Autodesk Fusion 360 part; units mm, degrees
note: some values were not read from the file. Chosen so that the rebuilt part matches the saved one: a direction. Set by a fixed rule: which sketch regions a step uses.
(part 3 of 8)
  spline S31 degree 5 poles (2.8779, -27.5468) (2.8797, -27.5528) (2.8833, -27.5648) (2.8888, -27.5828) (2.8962, -27.6068) (2.9055, -27.6366) (2.915, -27.6664) (2.9246, -27.6961) (2.9342, -27.7257) (2.944, -27.7552) (2.954, -27.7847) (2.964, -27.814) (2.9742, -27.8433) (2.9845, -27.8725) (2.9949, -27.9015) (3.0054, -27.9305) (3.0161, -27.9594) (3.0268, -27.9882) (3.0377, -28.017) (3.0487, -28.0456) (3.0599, -28.0741) (3.0711, -28.1025) (3.0825, -28.1309) (3.094, -28.1591) (3.1057, -28.1872) (3.1174, -28.2153) (3.1293, -28.2432) (3.1413, -28.271) (3.1535, -28.2987) (3.1657, -28.3264) (3.1781, -28.3539) (3.1907, -28.3813) (3.2033, -28.4086) (3.2161, -28.4357) (3.229, -28.4628) (3.2421, -28.4897) (3.2553, -28.5166) (3.2686, -28.5433) (3.2821, -28.5699) (3.2957, -28.5964) (3.3094, -28.6227) (3.3233, -28.6489) (3.3373, -28.675) (3.3515, -28.701) (3.3658, -28.7268) (3.3802, -28.7525) (3.3948, -28.7781) (3.4096, -28.8035) (3.4244, -28.8288) (3.4395, -28.854) (3.4547, -28.879) (3.47, -28.9038) (3.4856, -28.9285) (3.5013, -28.953) (3.5172, -28.9774) (3.5332, -29.0015) (3.5494, -29.0256) (3.5657, -29.0495) (3.5822, -29.0732) (3.5989, -29.0967) (3.6158, -29.12) (3.6329, -29.1431) (3.6504, -29.1659) (3.668, -29.1884) (3.686, -29.2107) (3.704, -29.2327) (3.7222, -29.2547) (3.7405, -29.2765) (3.759, -29.2981) (3.7779, -29.3193) (3.7972, -29.34) (3.8133, -29.3559) (3.8258, -29.3673) (3.8344, -29.3748) (3.8387, -29.3784) knots -1 -1 -1 -1 -1 -1 -0.98571429 -0.97142857 -0.95714286 -0.94285714 -0.92857143 -0.91428571 -0.9 -0.88571429 -0.87142857 -0.85714286 -0.84285714 -0.82857143 -0.81428571 -0.8 -0.78571429 -0.77142857 -0.75714286 -0.74285714 -0.72857143 -0.71428571 -0.7 -0.68571429 -0.67142857 -0.65714286 -0.64285714 -0.62857143 -0.61428571 -0.6 -0.58571429 -0.57142857 -0.55714286 -0.54285714 -0.52857143 -0.51428571 -0.5 -0.48571429 -0.47142857 -0.45714286 -0.44285714 -0.42857143 -0.41428571 -0.4 -0.38571429 -0.37142857 -0.35714286 -0.34285714 -0.32857143 -0.31428571 -0.3 -0.28571429 -0.27142857 -0.25714286 -0.24285714 -0.22857143 -0.21428571 -0.2 -0.18571429 -0.17142857 -0.15714286 -0.14285714 -0.12857143 -0.11428571 -0.1 -0.08571429 -0.07142857 -0.05714286 -0.04285714 -0.02857143 -0.01428571 0 0 0 0 0 0
  line L31 (3.8387, -29.3784) -> (4.1341, -29.6298)
  arc A63 (4.146, -29.7701) -> (4.1341, -29.6298) centre (4.0693, -29.706) ccw
  arc A64 (4.146, -29.7701) -> (3.5162, -30.5908) centre (13.5, -37.5997) ccw
  arc A65 (3.3776, -30.6157) -> (3.5162, -30.5908) centre (3.4344, -30.5334) ccw
  line L32 (3.3776, -30.6157) -> (3.0583, -30.3954)
  spline S32 degree 5 poles (3.0583, -30.3954) (3.0537, -30.3922) (3.0443, -30.3859) (3.03, -30.3768) (3.0105, -30.3653) (2.9855, -30.352) (2.9601, -30.3393) (2.9345, -30.327) (2.9087, -30.315) (2.8827, -30.3031) (2.8567, -30.2913) (2.8306, -30.2798) (2.8043, -30.2685) (2.7778, -30.2576) (2.751, -30.247) (2.7242, -30.2367) (2.6971, -30.2267) (2.6699, -30.2169) (2.6426, -30.2073) (2.6152, -30.1979) (2.5877, -30.1887) (2.5601, -30.1796) (2.5323, -30.1708) (2.5045, -30.1622) (2.4765, -30.1538) (2.4484, -30.1456) (2.4202, -30.1375) (2.392, -30.1297) (2.3636, -30.1221) (2.3351, -30.1146) (2.3065, -30.1073) (2.2779, -30.1001) (2.2491, -30.0932) (2.2203, -30.0864) (2.1914, -30.0798) (2.1624, -30.0733) (2.1333, -30.067) (2.1041, -30.0609) (2.0748, -30.055) (2.0455, -30.0492) (2.0161, -30.0435) (1.9866, -30.0381) (1.957, -30.0327) (1.9274, -30.0276) (1.8977, -30.0226) (1.8679, -30.0177) (1.8381, -30.013) (1.8082, -30.0085) (1.7782, -30.0041) (1.7481, -29.9998) (1.718, -29.9957) (1.6878, -29.9917) (1.6576, -29.9879) (1.6272, -29.9843) (1.5969, -29.9807) (1.5664, -29.9774) (1.5359, -29.9741) (1.5054, -29.971) (1.4748, -29.9681) (1.4441, -29.9653) (1.4134, -29.9626) (1.3826, -29.9601) (1.3517, -29.9577) (1.3208, -29.9555) (1.2899, -29.9534) (1.2589, -29.9514) (1.2278, -29.9496) (1.1967, -29.9479) (1.1656, -29.9463) (1.1343, -29.9449) (1.1031, -29.9436) (1.078, -29.9427) (1.0592, -29.942) (1.0467, -29.9416) (1.0404, -29.9415) knots 0 0 0 0 0 0 0.01428571 0.02857143 0.04285714 0.05714286 0.07142857 0.08571429 0.1 0.11428571 0.12857143 0.14285714 0.15714286 0.17142857 0.18571429 0.2 0.21428571 0.22857143 0.24285714 0.25714286 0.27142857 0.28571429 0.3 0.31428571 0.32857143 0.34285714 0.35714286 0.37142857 0.38571429 0.4 0.41428571 0.42857143 0.44285714 0.45714286 0.47142857 0.48571429 0.5 0.51428571 0.52857143 0.54285714 0.55714286 0.57142857 0.58571429 0.6 0.61428571 0.62857143 0.64285714 0.65714286 0.67142857 0.68571429 0.7 0.71428571 0.72857143 0.74285714 0.75714286 0.77142857 0.78571429 0.8 0.81428571 0.82857143 0.84285714 0.85714286 0.87142857 0.88571429 0.9 0.91428571 0.92857143 0.94285714 0.95714286 0.97142857 0.98571429 1 1 1 1 1 1
  arc A66 (1.0404, -29.9415) -> (0.638, -30.6385) centre (13.5, -37.5997) ccw
  spline S33 degree 5 poles (0.638, -30.6385) (0.6413, -30.6439) (0.6479, -30.6545) (0.6578, -30.6705) (0.6711, -30.6917) (0.6879, -30.7182) (0.7047, -30.7445) (0.7217, -30.7707) (0.7387, -30.7968) (0.7558, -30.8228) (0.773, -30.8486) (0.7903, -30.8744) (0.8077, -30.9) (0.8252, -30.9255) (0.8428, -30.9509) (0.8604, -30.9762) (0.8782, -31.0014) (0.8961, -31.0264) (0.914, -31.0513) (0.9321, -31.0761) (0.9502, -31.1008) (0.9684, -31.1253) (0.9868, -31.1498) (1.0052, -31.174) (1.0237, -31.1982) (1.0423, -31.2222) (1.061, -31.2461) (1.0798, -31.2699) (1.0988, -31.2935) (1.1178, -31.317) (1.1368, -31.3404) (1.156, -31.3636) (1.1753, -31.3867) (1.1947, -31.4096) (1.2142, -31.4324) (1.2338, -31.4551) (1.2535, -31.4776) (1.2733, -31.5) (1.2931, -31.5222) (1.3131, -31.5442) (1.3332, -31.5661) (1.3534, -31.5879) (1.3737, -31.6094) (1.3941, -31.6309) (1.4146, -31.6521) (1.4352, -31.6732) (1.4559, -31.6941) (1.4768, -31.7149) (1.4977, -31.7355) (1.5187, -31.7559) (1.5399, -31.7761) (1.5611, -31.7961) (1.5825, -31.8159) (1.6041, -31.8355) (1.6257, -31.8549) (1.6474, -31.8741) (1.6693, -31.8931) (1.6913, -31.912) (1.7133, -31.9306) (1.7355, -31.9491) (1.7579, -31.9672) (1.7804, -31.985) (1.8031, -32.0025) (1.826, -32.0197) (1.8491, -32.0366) (1.8723, -32.0532) (1.8955, -32.0697) (1.9189, -32.086) (1.9423, -32.1021) (1.966, -32.1178) (1.9901, -32.1327) (2.0097, -32.1439) (2.0248, -32.1517) (2.0349, -32.1567) (2.04, -32.1591) knots -1 -1 -1 -1 -1 -1 -0.98571429 -0.97142857 -0.95714286 -0.94285714 -0.92857143 -0.91428571 -0.9 -0.88571429 -0.87142857 -0.85714286 -0.84285714 -0.82857143 -0.81428571 -0.8 -0.78571429 -0.77142857 -0.75714286 -0.74285714 -0.72857143 -0.71428571 -0.7 -0.68571429 -0.67142857 -0.65714286 -0.64285714 -0.62857143 -0.61428571 -0.6 -0.58571429 -0.57142857 -0.55714286 -0.54285714 -0.52857143 -0.51428571 -0.5 -0.48571429 -0.47142857 -0.45714286 -0.44285714 -0.42857143 -0.41428571 -0.4 -0.38571429 -0.37142857 -0.35714286 -0.34285714 -0.32857143 -0.31428571 -0.3 -0.28571429 -0.27142857 -0.25714286 -0.24285714 -0.22857143 -0.21428571 -0.2 -0.18571429 -0.17142857 -0.15714286 -0.14285714 -0.12857143 -0.11428571 -0.1 -0.08571429 -0.07142857 -0.05714286 -0.04285714 -0.02857143 -0.01428571 0 0 0 0 0 0
  line L33 (2.04, -32.1591) -> (2.3904, -32.3255)
  arc A67 (2.4382, -32.4579) -> (2.3904, -32.3255) centre (2.3476, -32.4158) ccw
  arc A68 (2.4382, -32.4579) -> (2.0424, -33.4137) centre (13.5, -37.5997) ccw
  arc A69 (1.9149, -33.4735) -> (2.0424, -33.4137) centre (1.9484, -33.3793) ccw
  line L34 (1.9149, -33.4735) -> (1.5495, -33.3434)
  spline S34 degree 5 poles (1.5495, -33.3434) (1.5442, -33.3415) (1.5335, -33.3378) (1.5173, -33.3328) (1.4955, -33.3267) (1.4679, -33.3203) (1.4401, -33.3146) (1.4122, -33.3094) (1.3841, -33.3044) (1.356, -33.2996) (1.3278, -33.295) (1.2996, -33.2907) (1.2713, -33.2866) (1.2428, -33.2829) (1.2143, -33.2796) (1.1856, -33.2766) (1.1569, -33.2739) (1.1281, -33.2715) (1.0993, -33.2693) (1.0704, -33.2673) (1.0414, -33.2655) (1.0124, -33.2639) (0.9833, -33.2626) (0.9542, -33.2615) (0.925, -33.2606) (0.8957, -33.2599) (0.8664, -33.2595) (0.8371, -33.2592) (0.8077, -33.2592) (0.7782, -33.2593) (0.7488, -33.2597) (0.7192, -33.2602) (0.6897, -33.2609) (0.66, -33.2618) (0.6304, -33.2629) (0.6007, -33.2642) (0.571, -33.2656) (0.5412, -33.2673) (0.5114, -33.2691) (0.4816, -33.2711) (0.4517, -33.2733) (0.4218, -33.2756) (0.3919, -33.2781) (0.3619, -33.2808) (0.3319, -33.2836) (0.3019, -33.2867) (0.2719, -33.2898) (0.2418, -33.2932) (0.2117, -33.2967) (0.1815, -33.3004) (0.1514, -33.3042) (0.1212, -33.3082) (0.091, -33.3123) (0.0608, -33.3166) (0.0305, -33.3211) (0.0002, -33.3257) (-0.03, -33.3305) (-0.0604, -33.3354) (-0.0907, -33.3405) (-0.1211, -33.3457) (-0.1514, -33.3511) (-0.1818, -33.3566) (-0.2122, -33.3623) (-0.2427, -33.3681) (-0.2731, -33.3741) (-0.3036, -33.3802) (-0.334, -33.3865) (-0.3645, -33.3929) (-0.395, -33.3995) (-0.4255, -33.4062) (-0.4561, -33.413) (-0.4805, -33.4186) (-0.4988, -33.4229) (-0.511, -33.4257) (-0.5172, -33.4272) knots 0 0 0 0 0 0 0.01428571 0.02857143 0.04285714 0.05714286 0.07142857 0.08571429 0.1 0.11428571 0.12857143 0.14285714 0.15714286 0.17142857 0.18571429 0.2 0.21428571 0.22857143 0.24285714 0.25714286 0.27142857 0.28571429 0.3 0.31428571 0.32857143 0.34285714 0.35714286 0.37142857 0.38571429 0.4 0.41428571 0.42857143 0.44285714 0.45714286 0.47142857 0.48571429 0.5 0.51428571 0.52857143 0.54285714 0.55714286 0.57142857 0.58571429 0.6 0.61428571 0.62857143 0.64285714 0.65714286 0.67142857 0.68571429 0.7 0.71428571 0.72857143 0.74285714 0.75714286 0.77142857 0.78571429 0.8 0.81428571 0.82857143 0.84285714 0.85714286 0.87142857 0.88571429 0.9 0.91428571 0.92857143 0.94285714 0.95714286 0.97142857 0.98571429 1 1 1 1 1 1
  arc A70 (-0.5172, -33.4272) -> (-0.7255, -34.2047) centre (13.5, -37.5997) ccw
  spline S35 degree 5 poles (-0.7255, -34.2047) (-0.7209, -34.209) (-0.7118, -34.2176) (-0.698, -34.2304) (-0.6796, -34.2475) (-0.6566, -34.2687) (-0.6336, -34.2897) (-0.6104, -34.3107) (-0.5872, -34.3315) (-0.564, -34.3521) (-0.5406, -34.3726) (-0.5173, -34.393) (-0.4938, -34.4133) (-0.4703, -34.4334) (-0.4468, -34.4534) (-0.4232, -34.4733) (-0.3995, -34.493) (-0.3758, -34.5125) (-0.352, -34.5319) (-0.3281, -34.5512) (-0.3042, -34.5704) (-0.2803, -34.5894) (-0.2562, -34.6082) (-0.2321, -34.6269) (-0.208, -34.6454) (-0.1838, -34.6638) (-0.1595, -34.6821) (-0.1352, -34.7002) (-0.1108, -34.7181) (-0.0864, -34.7359) (-0.0619, -34.7535) (-0.0374, -34.771) (-0.0128, -34.7883) (0.0119, -34.8054) (0.0366, -34.8224) (0.0614, -34.8392) (0.0862, -34.8558) (0.1111, -34.8723) (0.1361, -34.8886) (0.1611, -34.9048) (0.1862, -34.9207) (0.2113, -34.9365) (0.2365, -34.9521) (0.2618, -34.9675) (0.2871, -34.9827) (0.3124, -34.9977) (0.3379, -35.0126) (0.3633, -35.0272) (0.3889, -35.0417) (0.4145, -35.056) (0.4401, -35.07) (0.4659, -35.0838) (0.4917, -35.0974) (0.5175, -35.1108) (0.5434, -35.124) (0.5694, -35.1369) (0.5954, -35.1496) (0.6215, -35.1621) (0.6477, -35.1744) (0.6739, -35.1865) (0.7002, -35.1982) (0.7266, -35.2096) (0.753, -35.2206) (0.7796, -35.2313) (0.8063, -35.2416) (0.833, -35.2517) (0.8597, -35.2616) (0.8865, -35.2713) (0.9133, -35.2808) (0.9402, -35.2898) (0.9673, -35.298) (0.9892, -35.3037) (1.0057, -35.3073) (1.0168, -35.3095) (1.0224, -35.3105) knots -1 -1 -1 -1 -1 -1 -0.98571429 -0.97142857 -0.95714286 -0.94285714 -0.92857143 -0.91428571 -0.9 -0.88571429 -0.87142857 -0.85714286 -0.84285714 -0.82857143 -0.81428571 -0.8 -0.78571429 -0.77142857 -0.75714286 -0.74285714 -0.72857143 -0.71428571 -0.7 -0.68571429 -0.67142857 -0.65714286 -0.64285714 -0.62857143 -0.61428571 -0.6 -0.58571429 -0.57142857 -0.55714286 -0.54285714 -0.52857143 -0.51428571 -0.5 -0.48571429 -0.47142857 -0.45714286 -0.44285714 -0.42857143 -0.41428571 -0.4 -0.38571429 -0.37142857 -0.35714286 -0.34285714 -0.32857143 -0.31428571 -0.3 -0.28571429 -0.27142857 -0.25714286 -0.24285714 -0.22857143 -0.21428571 -0.2 -0.18571429 -0.17142857 -0.15714286 -0.14285714 -0.12857143 -0.11428571 -0.1 -0.08571429 -0.07142857 -0.05714286 -0.04285714 -0.02857143 -0.01428571 0 0 0 0 0 0
  line L35 (1.0224, -35.3105) -> (1.4039, -35.3805)
  arc A71 (1.4844, -35.4961) -> (1.4039, -35.3805) centre (1.3859, -35.4789) ccw
  arc A72 (1.4844, -35.4961) -> (1.3493, -36.5217) centre (13.5, -37.5997) ccw
  arc A73 (1.2417, -36.6126) -> (1.3493, -36.5217) centre (1.2497, -36.5129) ccw
  line L36 (1.2417, -36.6126) -> (0.8551, -36.5815)
  spline S36 degree 5 poles (0.8551, -36.5815) (0.8494, -36.581) (0.8382, -36.5802) (0.8212, -36.5795) (0.7986, -36.5793) (0.7703, -36.5802) (0.742, -36.5819) (0.7136, -36.5841) (0.6853, -36.5866) (0.6569, -36.5893) (0.6285, -36.5921) (0.6001, -36.5952) (0.5716, -36.5986) (0.5432, -36.6024) (0.5148, -36.6066) (0.4863, -36.6111) (0.4579, -36.6159) (0.4295, -36.6211) (0.401, -36.6264) (0.3726, -36.632) (0.3441, -36.6377) (0.3157, -36.6437) (0.2873, -36.6499) (0.2588, -36.6564) (0.2304, -36.6631) (0.202, -36.67) (0.1736, -36.6772) (0.1451, -36.6845) (0.1167, -36.6921) (0.0883, -36.6999) (0.0599, -36.7078) (0.0316, -36.716) (0.0032, -36.7243) (-0.0252, -36.7328) (-0.0535, -36.7416) (-0.0819, -36.7505) (-0.1102, -36.7596) (-0.1385, -36.7689) (-0.1669, -36.7784) (-0.1952, -36.788) (-0.2234, -36.7978) (-0.2517, -36.8078) (-0.28, -36.818) (-0.3082, -36.8283) (-0.3365, -36.8389) (-0.3647, -36.8495) (-0.3929, -36.8604) (-0.4211, -36.8714) (-0.4492, -36.8826) (-0.4774, -36.8939) (-0.5055, -36.9054) (-0.5337, -36.9171) (-0.5618, -36.9289) (-0.5898, -36.9409) (-0.6179, -36.9531) (-0.646, -36.9653) (-0.674, -36.9778) (-0.702, -36.9904) (-0.73, -37.0032) (-0.7579, -37.0161) (-0.7859, -37.0291) (-0.8138, -37.0423) (-0.8417, -37.0557) (-0.8696, -37.0692) (-0.8975, -37.0828) (-0.9253, -37.0966) (-0.9531, -37.1106) (-0.9809, -37.1247) (-1.0087, -37.1389) (-1.0364, -37.1533) (-1.0641, -37.1678) (-1.0863, -37.1795) (-1.1029, -37.1884) (-1.1139, -37.1943) (-1.1195, -37.1973) knots 0 0 0 0 0 0 0.01428571 0.02857143 0.04285714 0.05714286 0.07142857 0.08571429 0.1 0.11428571 0.12857143 0.14285714 0.15714286 0.17142857 0.18571429 0.2 0.21428571 0.22857143 0.24285714 0.25714286 0.27142857 0.28571429 0.3 0.31428571 0.32857143 0.34285714 0.35714286 0.37142857 0.38571429 0.4 0.41428571 0.42857143 0.44285714 0.45714286 0.47142857 0.48571429 0.5 0.51428571 0.52857143 0.54285714 0.55714286 0.57142857 0.58571429 0.6 0.61428571 0.62857143 0.64285714 0.65714286 0.67142857 0.68571429 0.7 0.71428571 0.72857143 0.74285714 0.75714286 0.77142857 0.78571429 0.8 0.81428571 0.82857143 0.84285714 0.85714286 0.87142857 0.88571429 0.9 0.91428571 0.92857143 0.94285714 0.95714286 0.97142857 0.98571429 1 1 1 1 1 1
  arc A74 (-1.1195, -37.1973) -> (-1.1195, -38.0022) centre (13.5, -37.5997) ccw
  spline S37 degree 5 poles (-1.1195, -38.0022) (-1.1139, -38.0051) (-1.1029, -38.0111) (-1.0863, -38.0199) (-1.0641, -38.0317) (-1.0364, -38.0462) (-1.0087, -38.0605) (-0.9809, -38.0748) (-0.9531, -38.0889) (-0.9253, -38.1028) (-0.8975, -38.1166) (-0.8696, -38.1302) (-0.8417, -38.1437) (-0.8138, -38.1571) (-0.7859, -38.1703) (-0.7579, -38.1834) (-0.73, -38.1963) (-0.702, -38.209) (-0.674, -38.2216) (-0.646, -38.2341) (-0.6179, -38.2464) (-0.5898, -38.2585) (-0.5618, -38.2705) (-0.5337, -38.2823) (-0.5055, -38.294) (-0.4774, -38.3055) (-0.4492, -38.3168) (-0.4211, -38.328) (-0.3929, -38.339) (-0.3647, -38.3499) (-0.3365, -38.3606) (-0.3082, -38.3711) (-0.28, -38.3814) (-0.2517, -38.3916) (-0.2234, -38.4016) (-0.1952, -38.4114) (-0.1669, -38.4211) (-0.1385, -38.4305) (-0.1102, -38.4398) (-0.0819, -38.4489) (-0.0535, -38.4579) (-0.0252, -38.4666) (0.0032, -38.4751) (0.0316, -38.4835) (0.0599, -38.4916) (0.0883, -38.4996) (0.1167, -38.5073) (0.1451, -38.5149) (0.1736, -38.5223) (0.202, -38.5294) (0.2304, -38.5364) (0.2588, -38.5431) (0.2873, -38.5495) (0.3157, -38.5557) (0.3441, -38.5617) (0.3726, -38.5675) (0.401, -38.573) (0.4295, -38.5784) (0.4579, -38.5835) (0.4863, -38.5883) (0.5148, -38.5929) (0.5432, -38.5971) (0.5716, -38.6008) (0.6001, -38.6043) (0.6285, -38.6073) (0.6569, -38.6102) (0.6853, -38.6128) (0.7136, -38.6153) (0.742, -38.6175) (0.7703, -38.6192) (0.7986, -38.6201) (0.8212, -38.6199) (0.8382, -38.6192) (0.8494, -38.6184) (0.8551, -38.618) knots -1 -1 -1 -1 -1 -1 -0.98571429 -0.97142857 -0.95714286 -0.94285714 -0.92857143 -0.91428571 -0.9 -0.88571429 -0.87142857 -0.85714286 -0.84285714 -0.82857143 -0.81428571 -0.8 -0.78571429 -0.77142857 -0.75714286 -0.74285714 -0.72857143 -0.71428571 -0.7 -0.68571429 -0.67142857 -0.65714286 -0.64285714 -0.62857143 -0.61428571 -0.6 -0.58571429 -0.57142857 -0.55714286 -0.54285714 -0.52857143 -0.51428571 -0.5 -0.48571429 -0.47142857 -0.45714286 -0.44285714 -0.42857143 -0.41428571 -0.4 -0.38571429 -0.37142857 -0.35714286 -0.34285714 -0.32857143 -0.31428571 -0.3 -0.28571429 -0.27142857 -0.25714286 -0.24285714 -0.22857143 -0.21428571 -0.2 -0.18571429 -0.17142857 -0.15714286 -0.14285714 -0.12857143 -0.11428571 -0.1 -0.08571429 -0.07142857 -0.05714286 -0.04285714 -0.02857143 -0.01428571 0 0 0 0 0 0
  line L37 (0.8551, -38.618) -> (1.2417, -38.5868)
  arc A75 (1.3493, -38.6777) -> (1.2417, -38.5868) centre (1.2497, -38.6865) ccw
  arc A76 (1.3493, -38.6777) -> (1.4844, -39.7033) centre (13.5, -37.5997) ccw
  arc A77 (1.4039, -39.8189) -> (1.4844, -39.7033) centre (1.3859, -39.7205) ccw
  line L38 (1.4039, -39.8189) -> (1.0224, -39.8889)
  spline S38 degree 5 poles (1.0224, -39.8889) (1.0168, -39.8899) (1.0057, -39.8921) (0.9892, -39.8958) (0.9673, -39.9015) (0.9402, -39.9097) (0.9133, -39.9186) (0.8865, -39.9281) (0.8597, -39.9378) (0.833, -39.9477) (0.8063, -39.9578) (0.7796, -39.9682) (0.753, -39.9788) (0.7266, -39.9898) (0.7002, -40.0012) (0.6739, -40.013) (0.6477, -40.025) (0.6215, -40.0373) (0.5954, -40.0498) (0.5694, -40.0626) (0.5434, -40.0755) (0.5175, -40.0886) (0.4917, -40.102) (0.4659, -40.1156) (0.4401, -40.1294) (0.4145, -40.1435) (0.3889, -40.1577) (0.3633, -40.1722) (0.3379, -40.1869) (0.3124, -40.2017) (0.2871, -40.2167) (0.2618, -40.232) (0.2365, -40.2474) (0.2113, -40.2629) (0.1862, -40.2787) (0.1611, -40.2947) (0.1361, -40.3108) (0.1111, -40.3271) (0.0862, -40.3436) (0.0614, -40.3602) (0.0366, -40.377) (0.0119, -40.394) (-0.0128, -40.4112) (-0.0374, -40.4285) (-0.0619, -40.4459) (-0.0864, -40.4636) (-0.1108, -40.4813) (-0.1352, -40.4993) (-0.1595, -40.5174) (-0.1838, -40.5356) (-0.208, -40.554) (-0.2321, -40.5725) (-0.2562, -40.5912) (-0.2803, -40.6101) (-0.3042, -40.6291) (-0.3281, -40.6482) (-0.352, -40.6675) (-0.3758, -40.6869) (-0.3995, -40.7065) (-0.4232, -40.7262) (-0.4468, -40.746) (-0.4703, -40.766) (-0.4938, -40.7861) (-0.5173, -40.8064) (-0.5406, -40.8268) (-0.564, -40.8473) (-0.5872, -40.868) (-0.6104, -40.8888) (-0.6336, -40.9097) (-0.6566, -40.9308) (-0.6796, -40.952) (-0.698, -40.969) (-0.7118, -40.9819) (-0.7209, -40.9905) (-0.7255, -40.9948) knots 0 0 0 0 0 0 0.01428571 0.02857143 0.04285714 0.05714286 0.07142857 0.08571429 0.1 0.11428571 0.12857143 0.14285714 0.15714286 0.17142857 0.18571429 0.2 0.21428571 0.22857143 0.24285714 0.25714286 0.27142857 0.28571429 0.3 0.31428571 0.32857143 0.34285714 0.35714286 0.37142857 0.38571429 0.4 0.41428571 0.42857143 0.44285714 0.45714286 0.47142857 0.48571429 0.5 0.51428571 0.52857143 0.54285714 0.55714286 0.57142857 0.58571429 0.6 0.61428571 0.62857143 0.64285714 0.65714286 0.67142857 0.68571429 0.7 0.71428571 0.72857143 0.74285714 0.75714286 0.77142857 0.78571429 0.8 0.81428571 0.82857143 0.84285714 0.85714286 0.87142857 0.88571429 0.9 0.91428571 0.92857143 0.94285714 0.95714286 0.97142857 0.98571429 1 1 1 1 1 1
  arc A78 (-0.7255, -40.9948) -> (-0.5172, -41.7722) centre (13.5, -37.5997) ccw
  spline S39 degree 5 poles (-0.5172, -41.7722) (-0.511, -41.7737) (-0.4988, -41.7766) (-0.4805, -41.7808) (-0.4561, -41.7864) (-0.4255, -41.7933) (-0.395, -41.8) (-0.3645, -41.8065) (-0.334, -41.8129) (-0.3036, -41.8192) (-0.2731, -41.8253) (-0.2427, -41.8313) (-0.2122, -41.8371) (-0.1818, -41.8428) (-0.1514, -41.8483) (-0.1211, -41.8537) (-0.0907, -41.8589) (-0.0604, -41.864) (-0.03, -41.8689) (0.0002, -41.8737) (0.0305, -41.8783) (0.0608, -41.8828) (0.091, -41.8871) (0.1212, -41.8912) (0.1514, -41.8952) (0.1815, -41.8991) (0.2117, -41.9027) (0.2418, -41.9062) (0.2719, -41.9096) (0.3019, -41.9128) (0.3319, -41.9158) (0.3619, -41.9186) (0.3919, -41.9213) (0.4218, -41.9238) (0.4517, -41.9262) (0.4816, -41.9283) (0.5114, -41.9303) (0.5412, -41.9321) (0.571, -41.9338) (0.6007, -41.9353) (0.6304, -41.9365) (0.66, -41.9376) (0.6897, -41.9385) (0.7192, -41.9393) (0.7488, -41.9398) (0.7782, -41.9401) (0.8077, -41.9403) (0.8371, -41.9402) (0.8664, -41.94) (0.8957, -41.9395) (0.925, -41.9389) (0.9542, -41.938) (0.9833, -41.9369) (1.0124, -41.9355) (1.0414, -41.9339) (1.0704, -41.9321) (1.0993, -41.9301) (1.1281, -41.9279) (1.1569, -41.9255) (1.1856, -41.9228) (1.2143, -41.9199) (1.2428, -41.9165) (1.2713, -41.9128) (1.2996, -41.9088) (1.3278, -41.9044) (1.356, -41.8998) (1.3841, -41.895) (1.4122, -41.89) (1.4401, -41.8848) (1.4679, -41.8791) (1.4955, -41.8727) (1.5173, -41.8667) (1.5335, -41.8616) (1.5442, -41.8579) (1.5495, -41.856) knots -1 -1 -1 -1 -1 -1 -0.98571429 -0.97142857 -0.95714286 -0.94285714 -0.92857143 -0.91428571 -0.9 -0.88571429 -0.87142857 -0.85714286 -0.84285714 -0.82857143 -0.81428571 -0.8 -0.78571429 -0.77142857 -0.75714286 -0.74285714 -0.72857143 -0.71428571 -0.7 -0.68571429 -0.67142857 -0.65714286 -0.64285714 -0.62857143 -0.61428571 -0.6 -0.58571429 -0.57142857 -0.55714286 -0.54285714 -0.52857143 -0.51428571 -0.5 -0.48571429 -0.47142857 -0.45714286 -0.44285714 -0.42857143 -0.41428571 -0.4 -0.38571429 -0.37142857 -0.35714286 -0.34285714 -0.32857143 -0.31428571 -0.3 -0.28571429 -0.27142857 -0.25714286 -0.24285714 -0.22857143 -0.21428571 -0.2 -0.18571429 -0.17142857 -0.15714286 -0.14285714 -0.12857143 -0.11428571 -0.1 -0.08571429 -0.07142857 -0.05714286 -0.04285714 -0.02857143 -0.01428571 0 0 0 0 0 0
  line L39 (1.5495, -41.856) -> (1.9149, -41.7259)
  arc A79 (2.0424, -41.7858) -> (1.9149, -41.7259) centre (1.9484, -41.8201) ccw
  arc A80 (2.0424, -41.7858) -> (2.4382, -42.7415) centre (13.5, -37.5997) ccw
  arc A81 (2.3904, -42.874) -> (2.4382, -42.7415) centre (2.3476, -42.7836) ccw
  line L40 (2.3904, -42.874) -> (2.04, -43.0403)
  spline S40 degree 5 poles (2.04, -43.0403) (2.0349, -43.0428) (2.0248, -43.0477) (2.0097, -43.0556) (1.9901, -43.0667) (1.966, -43.0817) (1.9423, -43.0973) (1.9189, -43.1134) (1.8955, -43.1297) (1.8723, -43.1462) (1.8491, -43.1629) (1.826, -43.1797) (1.8031, -43.1969) (1.7804, -43.2144) (1.7579, -43.2322) (1.7355, -43.2504) (1.7133, -43.2688) (1.6913, -43.2874) (1.6693, -43.3063) (1.6474, -43.3253) (1.6257, -43.3445) (1.6041, -43.3639) (1.5825, -43.3835) (1.5611, -43.4033) (1.5399, -43.4234) (1.5187, -43.4436) (1.4977, -43.464) (1.4768, -43.4846) (1.4559, -43.5053) (1.4352, -43.5262) (1.4146, -43.5473) (1.3941, -43.5686) (1.3737, -43.59) (1.3534, -43.6116) (1.3332, -43.6333) (1.3131, -43.6552) (1.2931, -43.6773) (1.2733, -43.6995) (1.2535, -43.7218) (1.2338, -43.7443) (1.2142, -43.767) (1.1947, -43.7898) (1.1753, -43.8127) (1.156, -43.8358) (1.1368, -43.859) (1.1178, -43.8824) (1.0988, -43.9059) (1.0798, -43.9295) (1.061, -43.9533) (1.0423, -43.9772) (1.0237, -44.0012) (1.0052, -44.0254) (0.9868, -44.0497) (0.9684, -44.0741) (0.9502, -44.0986) (0.9321, -44.1233) (0.914, -44.1481) (0.8961, -44.173) (0.8782, -44.1981) (0.8604, -44.2232) (0.8428, -44.2485) (0.8252, -44.2739) (0.8077, -44.2994) (0.7903, -44.3251) (0.773, -44.3508) (0.7558, -44.3767) (0.7387, -44.4027) (0.7217, -44.4288) (0.7047, -44.455) (0.6879, -44.4813) (0.6711, -44.5077) (0.6578, -44.5289) (0.6479, -44.5449) (0.6413, -44.5556) (0.638, -44.5609) knots 0 0 0 0 0 0 0.01428571 0.02857143 0.04285714 0.05714286 0.07142857 0.08571429 0.1 0.11428571 0.12857143 0.14285714 0.15714286 0.17142857 0.18571429 0.2 0.21428571 0.22857143 0.24285714 0.25714286 0.27142857 0.28571429 0.3 0.31428571 0.32857143 0.34285714 0.35714286 0.37142857 0.38571429 0.4 0.41428571 0.42857143 0.44285714 0.45714286 0.47142857 0.48571429 0.5 0.51428571 0.52857143 0.54285714 0.55714286 0.57142857 0.58571429 0.6 0.61428571 0.62857143 0.64285714 0.65714286 0.67142857 0.68571429 0.7 0.71428571 0.72857143 0.74285714 0.75714286 0.77142857 0.78571429 0.8 0.81428571 0.82857143 0.84285714 0.85714286 0.87142857 0.88571429 0.9 0.91428571 0.92857143 0.94285714 0.95714286 0.97142857 0.98571429 1 1 1 1 1 1
  arc A82 (0.638, -44.5609) -> (1.0404, -45.258) centre (13.5, -37.5997) ccw
  spline S41 degree 5 poles (1.0404, -45.258) (1.0467, -45.2578) (1.0592, -45.2574) (1.078, -45.2568) (1.1031, -45.2558) (1.1343, -45.2546) (1.1656, -45.2531) (1.1967, -45.2516) (1.2278, -45.2499) (1.2589, -45.248) (1.2899, -45.2461) (1.3208, -45.244) (1.3517, -45.2417) (1.3826, -45.2393) (1.4134, -45.2368) (1.4441, -45.2341) (1.4748, -45.2313) (1.5054, -45.2284) (1.5359, -45.2253) (1.5664, -45.2221) (1.5969, -45.2187) (1.6272, -45.2152) (1.6576, -45.2115) (1.6878, -45.2077) (1.718, -45.2037) (1.7481, -45.1996) (1.7782, -45.1954) (1.8082, -45.191) (1.8381, -45.1864) (1.8679, -45.1817) (1.8977, -45.1769) (1.9274, -45.1719) (1.957, -45.1667) (1.9866, -45.1614) (2.0161, -45.1559) (2.0455, -45.1503) (2.0748, -45.1445) (2.1041, -45.1385) (2.1333, -45.1324) (2.1624, -45.1261) (2.1914, -45.1197) (2.2203, -45.113) (2.2491, -45.1063) (2.2779, -45.0993) (2.3065, -45.0922) (2.3351, -45.0849) (2.3636, -45.0774) (2.392, -45.0697) (2.4202, -45.0619) (2.4484, -45.0539) (2.4765, -45.0457) (2.5045, -45.0373) (2.5323, -45.0286) (2.5601, -45.0198) (2.5877, -45.0108) (2.6152, -45.0015) (2.6426, -44.9921) (2.6699, -44.9825) (2.6971, -44.9727) (2.7242, -44.9627) (2.751, -44.9524) (2.7778, -44.9418) (2.8043, -44.9309) (2.8306, -44.9196) (2.8567, -44.9081) (2.8827, -44.8964) (2.9087, -44.8845) (2.9345, -44.8724) (2.9601, -44.8601) (2.9855, -44.8475) (3.0105, -44.8341) (3.03, -44.8226) (3.0443, -44.8135) (3.0537, -44.8072) (3.0583, -44.804) knots -1 -1 -1 -1 -1 -1 -0.98571429 -0.97142857 -0.95714286 -0.94285714 -0.92857143 -0.91428571 -0.9 -0.88571429 -0.87142857 -0.85714286 -0.84285714 -0.82857143 -0.81428571 -0.8 -0.78571429 -0.77142857 -0.75714286 -0.74285714 -0.72857143 -0.71428571 -0.7 -0.68571429 -0.67142857 -0.65714286 -0.64285714 -0.62857143 -0.61428571 -0.6 -0.58571429 -0.57142857 -0.55714286 -0.54285714 -0.52857143 -0.51428571 -0.5 -0.48571429 -0.47142857 -0.45714286 -0.44285714 -0.42857143 -0.41428571 -0.4 -0.38571429 -0.37142857 -0.35714286 -0.34285714 -0.32857143 -0.31428571 -0.3 -0.28571429 -0.27142857 -0.25714286 -0.24285714 -0.22857143 -0.21428571 -0.2 -0.18571429 -0.17142857 -0.15714286 -0.14285714 -0.12857143 -0.11428571 -0.1 -0.08571429 -0.07142857 -0.05714286 -0.04285714 -0.02857143 -0.01428571 0 0 0 0 0 0
  line L41 (3.0583, -44.804) -> (3.3776, -44.5837)
  arc A83 (3.5162, -44.6086) -> (3.3776, -44.5837) centre (3.4344, -44.666) ccw
  arc A84 (3.5162, -44.6086) -> (4.146, -45.4293) centre (13.5, -37.5997) ccw
  arc A85 (4.1341, -45.5696) -> (4.146, -45.4293) centre (4.0693, -45.4935) ccw
  line L42 (4.1341, -45.5696) -> (3.8387, -45.821)
  spline S42 degree 5 poles (3.8387, -45.821) (3.8344, -45.8247) (3.8258, -45.8321) (3.8133, -45.8436) (3.7972, -45.8594) (3.7779, -45.8801) (3.759, -45.9013) (3.7405, -45.9229) (3.7222, -45.9447) (3.704, -45.9667) (3.686, -45.9888) (3.668, -46.011) (3.6504, -46.0335) (3.6329, -46.0563) (3.6158, -46.0794) (3.5989, -46.1027) (3.5822, -46.1262) (3.5657, -46.15) (3.5494, -46.1739) (3.5332, -46.1979) (3.5172, -46.2221) (3.5013, -46.2464) (3.4856, -46.2709) (3.47, -46.2956) (3.4547, -46.3204) (3.4395, -46.3454) (3.4244, -46.3706) (3.4096, -46.3959) (3.3948, -46.4213) (3.3802, -46.4469) (3.3658, -46.4726) (3.3515, -46.4984) (3.3373, -46.5244) (3.3233, -46.5505) (3.3094, -46.5767) (3.2957, -46.6031) (3.2821, -46.6295) (3.2686, -46.6561) (3.2553, -46.6829) (3.2421, -46.7097) (3.229, -46.7366) (3.2161, -46.7637) (3.2033, -46.7909) (3.1907, -46.8182) (3.1781, -46.8456) (3.1657, -46.8731) (3.1535, -46.9007) (3.1413, -46.9284) (3.1293, -46.9562) (3.1174, -46.9842) (3.1057, -47.0122) (3.094, -47.0403) (3.0825, -47.0686) (3.0711, -47.0969) (3.0599, -47.1253) (3.0487, -47.1538) (3.0377, -47.1825) (3.0268, -47.2112) (3.0161, -47.24) (3.0054, -47.2689) (2.9949, -47.2979) (2.9845, -47.327) (2.9742, -47.3561) (2.964, -47.3854) (2.954, -47.4148) (2.944, -47.4442) (2.9342, -47.4737) (2.9246, -47.5033) (2.915, -47.533) (2.9055, -47.5628) (2.8962, -47.5927) (2.8888, -47.6166) (2.8833, -47.6346) (2.8797, -47.6467) (2.8779, -47.6527) knots 0 0 0 0 0 0 0.01428571 0.02857143 0.04285714 0.05714286 0.07142857 0.08571429 0.1 0.11428571 0.12857143 0.14285714 0.15714286 0.17142857 0.18571429 0.2 0.21428571 0.22857143 0.24285714 0.25714286 0.27142857 0.28571429 0.3 0.31428571 0.32857143 0.34285714 0.35714286 0.37142857 0.38571429 0.4 0.41428571 0.42857143 0.44285714 0.45714286 0.47142857 0.48571429 0.5 0.51428571 0.52857143 0.54285714 0.55714286 0.57142857 0.58571429 0.6 0.61428571 0.62857143 0.64285714 0.65714286 0.67142857 0.68571429 0.7 0.71428571 0.72857143 0.74285714 0.75714286 0.77142857 0.78571429 0.8 0.81428571 0.82857143 0.84285714 0.85714286 0.87142857 0.88571429 0.9 0.91428571 0.92857143 0.94285714 0.95714286 0.97142857 0.98571429 1 1 1 1 1 1
  arc A86 (2.8779, -47.6527) -> (3.4471, -48.2218) centre (13.5, -37.5997) ccw
  spline S43 degree 5 poles (3.4471, -48.2218) (3.4531, -48.22) (3.4651, -48.2164) (3.4831, -48.2109) (3.507, -48.2035) (3.5369, -48.1942) (3.5667, -48.1847) (3.5964, -48.1752) (3.626, -48.1655) (3.6555, -48.1557) (3.685, -48.1457) (3.7143, -48.1357) (3.7436, -48.1255) (3.7727, -48.1152) (3.8018, -48.1048) (3.8308, -48.0943) (3.8597, -48.0837) (3.8885, -48.0729) (3.9172, -48.062) (3.9459, -48.051) (3.9744, -48.0398) (4.0028, -48.0286) (4.0312, -48.0172) (4.0594, -48.0057) (4.0875, -47.994) (4.1155, -47.9823) (4.1435, -47.9704) (4.1713, -47.9584) (4.199, -47.9462) (4.2266, -47.934) (4.2541, -47.9216) (4.2815, -47.909) (4.3088, -47.8964) (4.336, -47.8836) (4.3631, -47.8707) (4.39, -47.8576) (4.4169, -47.8444) (4.4436, -47.8311) (4.4702, -47.8176) (4.4967, -47.804) (4.523, -47.7903) (4.5492, -47.7764) (4.5753, -47.7624) (4.6013, -47.7483) (4.6271, -47.7339) (4.6528, -47.7195) (4.6784, -47.7049) (4.7038, -47.6902) (4.7291, -47.6753) (4.7543, -47.6602) (4.7793, -47.645) (4.8041, -47.6297) (4.8288, -47.6141) (4.8533, -47.5984) (4.8776, -47.5825) (4.9018, -47.5665) (4.9259, -47.5503) (4.9497, -47.534) (4.9735, -47.5175) (4.997, -47.5008) (5.0203, -47.4839) (5.0434, -47.4668) (5.0662, -47.4494) (5.0887, -47.4317) (5.1109, -47.4138) (5.133, -47.3957) (5.155, -47.3775) (5.1768, -47.3592) (5.1984, -47.3407) (5.2196, -47.3218) (5.2403, -47.3025) (5.2561, -47.2864) (5.2676, -47.2739) (5.275, -47.2654) (5.2787, -47.261) knots -1 -1 -1 -1 -1 -1 -0.98571429 -0.97142857 -0.95714286 -0.94285714 -0.92857143 -0.91428571 -0.9 -0.88571429 -0.87142857 -0.85714286 -0.84285714 -0.82857143 -0.81428571 -0.8 -0.78571429 -0.77142857 -0.75714286 -0.74285714 -0.72857143 -0.71428571 -0.7 -0.68571429 -0.67142857 -0.65714286 -0.64285714 -0.62857143 -0.61428571 -0.6 -0.58571429 -0.57142857 -0.55714286 -0.54285714 -0.52857143 -0.51428571 -0.5 -0.48571429 -0.47142857 -0.45714286 -0.44285714 -0.42857143 -0.41428571 -0.4 -0.38571429 -0.37142857 -0.35714286 -0.34285714 -0.32857143 -0.31428571 -0.3 -0.28571429 -0.27142857 -0.25714286 -0.24285714 -0.22857143 -0.21428571 -0.2 -0.18571429 -0.17142857 -0.15714286 -0.14285714 -0.12857143 -0.11428571 -0.1 -0.08571429 -0.07142857 -0.05714286 -0.04285714 -0.02857143 -0.01428571 0 0 0 0 0 0
  line L43 (5.2787, -47.261) -> (5.5301, -46.9656)
  arc A87 (5.6704, -46.9538) -> (5.5301, -46.9656) centre (5.6062, -47.0304) ccw
  arc A88 (5.6704, -46.9538) -> (6.4911, -47.5835) centre (13.5, -37.5997) ccw
  arc A89 (6.516, -47.7221) -> (6.4911, -47.5835) centre (6.4337, -47.6653) ccw
  line L44 (6.516, -47.7221) -> (6.2957, -48.0414)
  spline S44 degree 5 poles (6.2957, -48.0414) (6.2925, -48.0461) (6.2862, -48.0554) (6.2771, -48.0698) (6.2656, -48.0893) (6.2523, -48.1142) (6.2396, -48.1396) (6.2273, -48.1653) (6.2152, -48.1911) (6.2033, -48.217) (6.1916, -48.243) (6.1801, -48.2691) (6.1688, -48.2954) (6.1579, -48.322) (6.1473, -48.3487) (6.137, -48.3756) (6.127, -48.4026) (6.1172, -48.4298) (6.1076, -48.4571) (6.0982, -48.4845) (6.089, -48.512) (6.0799, -48.5396) (6.0711, -48.5674) (6.0625, -48.5952) (6.0541, -48.6232) (6.0458, -48.6513) (6.0378, -48.6795) (6.03, -48.7078) (6.0223, -48.7361) (6.0149, -48.7646) (6.0076, -48.7932) (6.0004, -48.8218) (5.9935, -48.8506) (5.9867, -48.8794) (5.9801, -48.9083) (5.9736, -48.9374) (5.9673, -48.9665) (5.9612, -48.9956) (5.9553, -49.0249) (5.9495, -49.0542) (5.9438, -49.0836) (5.9383, -49.1131) (5.933, -49.1427) (5.9279, -49.1723) (5.9229, -49.202) (5.918, -49.2318) (5.9133, -49.2616) (5.9087, -49.2916) (5.9043, -49.3216) (5.9001, -49.3516) (5.896, -49.3817) (5.892, -49.4119) (5.8882, -49.4422) (5.8845, -49.4725) (5.881, -49.5028) (5.8776, -49.5333) (5.8744, -49.5638) (5.8713, -49.5943) (5.8684, -49.625) (5.8656, -49.6556) (5.8629, -49.6864) (5.8604, -49.7171) (5.858, -49.748) (5.8558, -49.7789) (5.8536, -49.8098) (5.8517, -49.8408) (5.8498, -49.8719) (5.8481, -49.903) (5.8466, -49.9342) (5.8452, -49.9654) (5.8439, -49.9966) (5.843, -50.0217) (5.8423, -50.0405) (5.8419, -50.053) (5.8417, -50.0593) knots 0 0 0 0 0 0 0.01428571 0.02857143 0.04285714 0.05714286 0.07142857 0.08571429 0.1 0.11428571 0.12857143 0.14285714 0.15714286 0.17142857 0.18571429 0.2 0.21428571 0.22857143 0.24285714 0.25714286 0.27142857 0.28571429 0.3 0.31428571 0.32857143 0.34285714 0.35714286 0.37142857 0.38571429 0.4 0.41428571 0.42857143 0.44285714 0.45714286 0.47142857 0.48571429 0.5 0.51428571 0.52857143 0.54285714 0.55714286 0.57142857 0.58571429 0.6 0.61428571 0.62857143 0.64285714 0.65714286 0.67142857 0.68571429 0.7 0.71428571 0.72857143 0.74285714 0.75714286 0.77142857 0.78571429 0.8 0.81428571 0.82857143 0.84285714 0.85714286 0.87142857 0.88571429 0.9 0.91428571 0.92857143 0.94285714 0.95714286 0.97142857 0.98571429 1 1 1 1 1 1
  arc A90 (5.8417, -50.0593) -> (6.5388, -50.4618) centre (13.5, -37.5997) ccw
  spline S45 degree 5 poles (6.5388, -50.4618) (6.5441, -50.4585) (6.5548, -50.4518) (6.5708, -50.4419) (6.592, -50.4286) (6.6184, -50.4118) (6.6448, -50.395) (6.671, -50.3781) (6.6971, -50.361) (6.723, -50.3439) (6.7489, -50.3267) (6.7747, -50.3094) (6.8003, -50.292) (6.8258, -50.2745) (6.8512, -50.257) (6.8765, -50.2393) (6.9017, -50.2215) (6.9267, -50.2037) (6.9516, -50.1857) (6.9764, -50.1677) (7.0011, -50.1495) (7.0256, -50.1313) (7.05, -50.1129) (7.0743, -50.0945) (7.0985, -50.076) (7.1225, -50.0574) (7.1464, -50.0387) (7.1702, -50.0199) (7.1938, -50.001) (7.2173, -49.982) (7.2407, -49.9629) (7.2639, -49.9437) (7.287, -49.9244) (7.3099, -49.905) (7.3327, -49.8855) (7.3554, -49.8659) (7.3779, -49.8462) (7.4002, -49.8265) (7.4225, -49.8066) (7.4445, -49.7866) (7.4664, -49.7665) (7.4881, -49.7463) (7.5097, -49.726) (7.5311, -49.7056) (7.5524, -49.6851) (7.5735, -49.6645) (7.5944, -49.6438) (7.6152, -49.623) (7.6357, -49.602) (7.6561, -49.581) (7.6764, -49.5598) (7.6964, -49.5386) (7.7162, -49.5172) (7.7358, -49.4957) (7.7552, -49.474) (7.7744, -49.4523) (7.7934, -49.4304) (7.8123, -49.4085) (7.8309, -49.3864) (7.8493, -49.3642) (7.8675, -49.3418) (7.8853, -49.3193) (7.9028, -49.2966) (7.92, -49.2737) (7.9369, -49.2506) (7.9535, -49.2274) (7.97, -49.2042) (7.9863, -49.1808) (8.0024, -49.1574) (8.0181, -49.1337) (8.033, -49.1096) (8.0441, -49.09) (8.052, -49.0749) (8.057, -49.0648) (8.0594, -49.0597) knots -1 -1 -1 -1 -1 -1 -0.98571429 -0.97142857 -0.95714286 -0.94285714 -0.92857143 -0.91428571 -0.9 -0.88571429 -0.87142857 -0.85714286 -0.84285714 -0.82857143 -0.81428571 -0.8 -0.78571429 -0.77142857 -0.75714286 -0.74285714 -0.72857143 -0.71428571 -0.7 -0.68571429 -0.67142857 -0.65714286 -0.64285714 -0.62857143 -0.61428571 -0.6 -0.58571429 -0.57142857 -0.55714286 -0.54285714 -0.52857143 -0.51428571 -0.5 -0.48571429 -0.47142857 -0.45714286 -0.44285714 -0.42857143 -0.41428571 -0.4 -0.38571429 -0.37142857 -0.35714286 -0.34285714 -0.32857143 -0.31428571 -0.3 -0.28571429 -0.27142857 -0.25714286 -0.24285714 -0.22857143 -0.21428571 -0.2 -0.18571429 -0.17142857 -0.15714286 -0.14285714 -0.12857143 -0.11428571 -0.1 -0.08571429 -0.07142857 -0.05714286 -0.04285714 -0.02857143 -0.01428571 0 0 0 0 0 0
  line L45 (8.0594, -49.0597) -> (8.2257, -48.7093)
  arc A91 (8.3582, -48.6615) -> (8.2257, -48.7093) centre (8.3161, -48.7522) ccw
  arc A92 (8.3582, -48.6615) -> (9.3139, -49.0573) centre (13.5, -37.5997) ccw
  arc A93 (9.3738, -49.1848) -> (9.3139, -49.0573) centre (9.2796, -49.1513) ccw
  line L46 (9.3738, -49.1848) -> (9.2437, -49.5502)
  spline S46 degree 5 poles (9.2437, -49.5502) (9.2418, -49.5556) (9.2381, -49.5663) (9.233, -49.5824) (9.227, -49.6042) (9.2206, -49.6318) (9.2149, -49.6596) (9.2097, -49.6876) (9.2047, -49.7156) (9.1999, -49.7437) (9.1953, -49.7719) (9.1909, -49.8001) (9.1869, -49.8284) (9.1832, -49.8569) (9.1799, -49.8854) (9.1769, -49.9141) (9.1742, -49.9428) (9.1718, -49.9716) (9.1696, -50.0004) (9.1676, -50.0294) (9.1658, -50.0583) (9.1642, -50.0873) (9.1629, -50.1164) (9.1617, -50.1455) (9.1609, -50.1747) (9.1602, -50.204) (9.1597, -50.2333) (9.1595, -50.2626) (9.1595, -50.292) (9.1596, -50.3215) (9.1599, -50.351) (9.1605, -50.3805) (9.1612, -50.4101) (9.1621, -50.4397) (9.1632, -50.4693) (9.1645, -50.499) (9.1659, -50.5287) (9.1676, -50.5585) (9.1694, -50.5883) (9.1714, -50.6181) (9.1736, -50.648) (9.1759, -50.6779) (9.1784, -50.7078) (9.1811, -50.7378) (9.1839, -50.7678) (9.1869, -50.7978) (9.1901, -50.8279) (9.1935, -50.8579) (9.197, -50.888) (9.2007, -50.9182) (9.2045, -50.9483) (9.2085, -50.9785) (9.2126, -51.0087) (9.2169, -51.0389) (9.2214, -51.0692) (9.226, -51.0995) (9.2308, -51.1298) (9.2357, -51.1601) (9.2408, -51.1904) (9.246, -51.2208) (9.2514, -51.2511) (9.2569, -51.2815) (9.2626, -51.3119) (9.2684, -51.3424) (9.2744, -51.3728) (9.2805, -51.4033) (9.2868, -51.4337) (9.2932, -51.4642) (9.2998, -51.4947) (9.3065, -51.5252) (9.3133, -51.5558) (9.3189, -51.5802) (9.3232, -51.5985) (9.326, -51.6108) (9.3275, -51.6169) knots 0 0 0 0 0 0 0.01428571 0.02857143 0.04285714 0.05714286 0.07142857 0.08571429 0.1 0.11428571 0.12857143 0.14285714 0.15714286 0.17142857 0.18571429 0.2 0.21428571 0.22857143 0.24285714 0.25714286 0.27142857 0.28571429 0.3 0.31428571 0.32857143 0.34285714 0.35714286 0.37142857 0.38571429 0.4 0.41428571 0.42857143 0.44285714 0.45714286 0.47142857 0.48571429 0.5 0.51428571 0.52857143 0.54285714 0.55714286 0.57142857 0.58571429 0.6 0.61428571 0.62857143 0.64285714 0.65714286 0.67142857 0.68571429 0.7 0.71428571 0.72857143 0.74285714 0.75714286 0.77142857 0.78571429 0.8 0.81428571 0.82857143 0.84285714 0.85714286 0.87142857 0.88571429 0.9 0.91428571 0.92857143 0.94285714 0.95714286 0.97142857 0.98571429 1 1 1 1 1 1
  arc A94 (9.3275, -51.6169) -> (10.1049, -51.8252) centre (13.5, -37.5997) ccw
  spline S47 degree 5 poles (10.1049, -51.8252) (10.1092, -51.8206) (10.1178, -51.8115) (10.1307, -51.7977) (10.1478, -51.7794) (10.1689, -51.7563) (10.19, -51.7333) (10.2109, -51.7101) (10.2317, -51.6869) (10.2524, -51.6637) (10.2729, -51.6404) (10.2933, -51.617) (10.3136, -51.5936) (10.3337, -51.5701) (10.3537, -51.5465) (10.3735, -51.5229) (10.3932, -51.4992) (10.4128, -51.4755) (10.4322, -51.4517) (10.4515, -51.4278) (10.4706, -51.4039) (10.4896, -51.38) (10.5085, -51.3559) (10.5272, -51.3319) (10.5457, -51.3077) (10.5641, -51.2835) (10.5824, -51.2593) (10.6004, -51.2349) (10.6184, -51.2106) (10.6362, -51.1861) (10.6538, -51.1616) (10.6713, -51.1371) (10.6886, -51.1125) (10.7057, -51.0878) (10.7227, -51.0631) (10.7395, -51.0383) (10.7561, -51.0135) (10.7726, -50.9886) (10.7889, -50.9636) (10.805, -50.9386) (10.821, -50.9135) (10.8368, -50.8884) (10.8524, -50.8632) (10.8678, -50.838) (10.883, -50.8127) (10.898, -50.7873) (10.9129, -50.7619) (10.9275, -50.7364) (10.942, -50.7108) (10.9562, -50.6852) (10.9703, -50.6596) (10.9841, -50.6339) (10.9977, -50.6081) (11.0111, -50.5822) (11.0242, -50.5563) (11.0372, -50.5303) (11.0499, -50.5043) (11.0624, -50.4782) (11.0747, -50.452) (11.0868, -50.4258) (11.0985, -50.3995) (11.1099, -50.3731) (11.1209, -50.3467) (11.1316, -50.3201) (11.1419, -50.2935) (11.152, -50.2668) (11.1619, -50.24) (11.1716, -50.2133) (11.1811, -50.1864) (11.1901, -50.1595) (11.1982, -50.1324) (11.2039, -50.1105) (11.2076, -50.094) (11.2098, -50.0829) (11.2108, -50.0773) knots -1 -1 -1 -1 -1 -1 -0.98571429 -0.97142857 -0.95714286 -0.94285714 -0.92857143 -0.91428571 -0.9 -0.88571429 -0.87142857 -0.85714286 -0.84285714 -0.82857143 -0.81428571 -0.8 -0.78571429 -0.77142857 -0.75714286 -0.74285714 -0.72857143 -0.71428571 -0.7 -0.68571429 -0.67142857 -0.65714286 -0.64285714 -0.62857143 -0.61428571 -0.6 -0.58571429 -0.57142857 -0.55714286 -0.54285714 -0.52857143 -0.51428571 -0.5 -0.48571429 -0.47142857 -0.45714286 -0.44285714 -0.42857143 -0.41428571 -0.4 -0.38571429 -0.37142857 -0.35714286 -0.34285714 -0.32857143 -0.31428571 -0.3 -0.28571429 -0.27142857 -0.25714286 -0.24285714 -0.22857143 -0.21428571 -0.2 -0.18571429 -0.17142857 -0.15714286 -0.14285714 -0.12857143 -0.11428571 -0.1 -0.08571429 -0.07142857 -0.05714286 -0.04285714 -0.02857143 -0.01428571 0 0 0 0 0 0
  line L47 (11.2108, -50.0773) -> (11.2808, -49.6958)
  arc A95 (11.3964, -49.6153) -> (11.2808, -49.6958) centre (11.3792, -49.7138) ccw
  circle A96 centre (13.5, -37.5997) radius 1.5
  line L48 (9.5, -37.5997) -> (9.5, -68.5997)
  arc A97 (9.5, -68.5997) -> (17.5, -68.5997) centre (13.5, -68.5997) ccw
  line L49 (17.5, -68.5997) -> (17.5, -37.5997)
  arc A98 (17.5, -37.5997) -> (9.5, -37.5997) centre (13.5, -37.5997) ccw
  line L50 (13.5, -37.5997) -> (13.5, -68.5997) construction
  circle A99 centre (13.5, -68.5997) radius 1.5
  dimension "d65" = 31
  dimension "d66" = 4
  dimension "d67" = 3
  constraint tangent L48 A97
  constraint tangent A97 L49
  constraint parallel L48 L49
  constraint tangent L49 A98
  constraint tangent L48 A98
  constraint vertical L50
  constraint coincident A0.centre A2.centre
  constraint concentric A97 A99
  measures "d65" distance of A0.centre A97.centre
  measures "d66" radius of A97
  measures "d67" diameter of A99
extrude "Extrude3" add sketch "Sketch5" against normal blind 3 contours A0 A1 L0 S0 A2 S1 L1 A3 A4 A5 L2 S2 A6 A94 S47 L47 A95 L48 L49 A98 | A0 A1 L0 S0 A2 S1 L1 A3 A4 A5 L2 S2 A6 A94 S47 L47 A95 L48 A97 L49 sketch seen with x (0, -1, 0) y (0, 0, 1) z (-1, 0, 0) at (-37.5997, -13.5, -3) bodies 5 in component "Spur Gear 24 teeth"